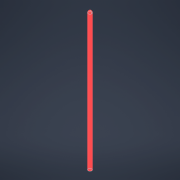
# Autodesk Inventor part: Blade
Saved by Autodesk Inventor 2022 (Build 260153000, 153)
## iProperties
Created: 2024-05-08
Part Number: Blade
Material: Generic
Document SubType Name: Modeling
Designer: jo_ki
Density: 1 g/cm^3
Appearance: Saber Blade
Author: jo_ki
Autodesk Inventor part; units mm, degrees
ref_plane "YZ Plane" through (0, 0, 0) normal (1, 0, 0) x (0, 1, 0)
ref_plane "XZ Plane" through (0, 0, 0) normal (0, 1, 0) x (-1, 0, 0)
ref_plane "XY Plane" through (0, 0, 0) normal (0, 0, 1) x (1, 0, 0)
sketch "Sketch1" plane through (0, 0, 0) normal (0, 0, 1) x (1, 0, 0)
  line L0 (-12.7, -457.2) -> (12.7, -457.2)
  line L1 (12.7, -457.2) -> (12.7, 457.2)
  line L2 (12.7, 457.2) -> (-12.7, 457.2)
  line L3 (-12.7, 457.2) -> (-12.7, -457.2)
  line L4 (-12.7, -457.2) -> (12.7, 457.2) construction
  line L5 (12.7, -457.2) -> (-12.7, 457.2) construction
  ellipse E0 centre (0, 442.2) end of major axis (0, 457.2) minor radius 12.7
  line L6 (10.7, -457.2) -> (10.7, 442.2)
  line L7 (-10.7, 442.2) -> (-10.7, -457.2)
  line L8 (0, -644.74) -> (0, 668.0398) construction
  ellipse E1 centre (0, 442.2) end of major axis (10.7, 442.2) minor radius 13
  line L9 (0, 455.2) -> (0, 429.2)
  line L10 (0, 457.2) -> (0, 455.2)
  line L11 (-11.1125, 480.4999) -> (11.1125, 480.4999)
  line L12 (11.1125, 480.4999) -> (11.1125, 476.7557)
  line L13 (11.1125, 476.7557) -> (-11.1125, 476.7557)
  line L14 (-11.1125, 476.7557) -> (-11.1125, 480.4999)
  line L15 (-11.1125, 480.4999) -> (11.1125, 476.7557) construction
  line L16 (11.1125, 480.4999) -> (-11.1125, 476.7557) construction
  line L17 (-12.7, 476.0898) -> (12.7, 476.0898)
  line L18 (12.7, 476.0898) -> (12.7, 472.3457)
  line L19 (12.7, 472.3457) -> (-12.7, 472.3457)
  line L20 (-12.7, 472.3457) -> (-12.7, 476.0898)
  line L21 (-12.7, 476.0898) -> (12.7, 472.3457) construction
  line L22 (12.7, 476.0898) -> (-12.7, 472.3457) construction
  point P0 (0, 0)
  point P1 (12.7, 442.2)
  point P2 (0, 478.6278)
  point P3 (0, 474.2178)
  dimension "d0" = 25.4
  dimension "d1" = 914.4
  dimension "d2" = 15
  dimension "d4" = 2
  dimension "d5" = 2
  dimension "d7" = 22.225
  dimension "d8" = 25.4
  constraints: 44 end point, 8 parallel, 7 point on line, 6 midpoint, 4 horizontal, 4 perpendicular, 3 vertical, 1 coincident, 1 collinear, 9 other
  measures "d0" distance of L1.end L2.end
  measures "d1" distance of L0.end L1.end
  measures "d2" distance from line of L2 point (0, 442.2)
  measures "d4" distance between parallel lines of L3 L7
  measures "d5" distance from line of L2 L9.start
  measures "d7" distance of L11.start L11.end
  measures "d8" distance between parallel lines of L20 L18
revolve "Revolution1" add sketch "Sketch1" angle 360 about axis through (0, -10, 0) along (0, 1, 0) contours L6 E0 L1 L0 | E0 L6 E1 L10
body "Solid1"
